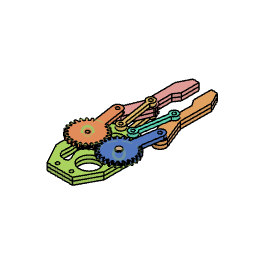
stage 3 v3 (Autodesk Fusion 360 design; units mm, degrees)
description: Spur Gear; Module: 1.125; Num Teeth: 24; Pressure Angle: 20.0; Backlash: 0.00 mm
Autodesk Fusion 360 part; units mm, degrees
note: some values were not read from the file. Chosen so that the rebuilt part matches the saved one: a direction. Set by a fixed rule: which sketch regions a step uses.
(part 1 of 6)
sketch "Sketch1" plane through (0, 0, 0) normal (0, 0, 1) x (1, 0, 0)
  line L0 (0, -5) -> (22, -5)
  arc A0 (22, -5) -> (22, 5) centre (22, 0) ccw
  line L1 (22, 5) -> (0, 5)
  arc A1 (0, 5) -> (0, -5) centre (0, 0) ccw
  line L2 (0, 0) -> (22, 0) construction
  circle A2 centre (0, 0) radius 1.5
  line L3 (20.05, 5) -> (54.05, 18.9791)
  line L4 (54.05, 18.9791) -> (57.9654, 9.456)
  line L5 (57.9654, 9.456) -> (23.1073, -4.8758)
  line L6 (44.6879, 15.1299) -> (56.0077, 14.2176)
  line L7 (43.85, 3.6525) -> (38, 5)
  line L8 (38, 5) -> (26.978, 0.4683)
  circle A3 centre (22, 0) radius 1.5
  dimension "d1" = 22
  dimension "d2" = 10
  dimension "d3" = 3
  dimension "d4" = 157.65
  dimension "d5" = 34
  dimension "d6" = 1.95
  dimension "d7" = 3
  constraint tangent L0 A0
  constraint tangent A0 L1
  constraint parallel L0 L1
  constraint tangent L1 A1
  constraint tangent L0 A1
  constraint horizontal L2
  constraint coincident A1.centre L2.start
  constraint coincident L1 L3.start
  constraint perpendicular L3 L4
  constraint coincident A0 L5.end
  constraint perpendicular L4 L5
  constraint coincident L3 L6.start
  constraint midpoint L4 L6.end
  constraint coincident L5 L7.start
  constraint coincident A0 L8.end
  constraint parallel L5 L8
  constraint concentric A0 A3
  measures "d1" distance of A1.centre A0.centre
  measures "d2" diameter of A1
  measures "d3" diameter of A2
  measures "d4" angle of L1 L3
  measures "d5" horizontal distance of L3.start L3.end
  measures "d6" horizontal distance of A0.centre L3.start
  measures "d7" diameter of A3
extrude "Extrude1" add sketch "Sketch1" along normal blind 3 contours L0 A0 L1 A1 L5 | A0 L1 L3 L4 L5 L6 L7 L8 makes body 1 in component "Component"
sketch "Sketch2" plane through (0, 0, 0) normal (0, 0, 1) x (1, 0, 0)
  circle A0 centre (75, 75) radius 1.5
  circle A1 centre (75, 75) radius 3.5
  circle A2 centre (106, 75) radius 3.5
  circle A3 centre (106, 75) radius 1.5
  line L0 (75, 75) -> (106, 75)
  line L1 (78.1623, 76.5) -> (102.8377, 76.5)
  line L2 (78.1623, 73.5) -> (102.8377, 73.5)
  dimension "d12" = 3
  dimension "d13" = 7
  dimension "d15" = 3
  dimension "d16" = 7
  dimension "d17" = 31
  dimension "d18" = 1.5
  constraint concentric A0 A1
  constraint concentric A2 A3
  constraint coincident A0.centre A1.centre
  constraint coincident A2.centre A3.centre
  constraint horizontal L0
  constraint coincident A1 L1.start
  constraint coincident A2 L1.end
  constraint parallel L0 L1
  constraint symmetric L0 L1.start L2.start
  constraint symmetric L0 L1.end L2.end
  measures "d12" diameter of A0
  measures "d13" diameter of A1
  measures "d15" diameter of A3
  measures "d16" diameter of A2
  measures "d17" distance of A0.centre A2.centre
  measures "d18" distance of L0 L1
extrude "Extrude1'" add sketch "Sketch2" along normal blind 3 separate body makes body 2 in component "Component'"
sketch "Sketch3" plane through (0, 0, 0) normal (0, 0, 1) x (1, 0, 0)
  line L0 (0, 0) -> (0, 62)
  line L1 (0, 62) -> (-7.9898, 62)
  line L2 (-7.9898, 62) -> (-20.5, 47.8997)
  line L3 (-20.5, 47.8997) -> (-20.5, 17.5997)
  line L4 (-20.5, 17.5997) -> (-11, 0)
  line L5 (-11, 0) -> (0, 0)
  circle A0 centre (-6, 4) radius 1.5
  circle A1 centre (-13.5, 37.5997) radius 1.5
  circle A2 centre (-5.2398, 58) radius 1.5
  line L6 (20.5, 17.5997) -> (11, 0)
  circle A3 centre (6, 4) radius 1.5
  circle A4 centre (13.5, 37.5997) radius 1.5
  line L7 (20.5, 47.8997) -> (20.5, 17.5997)
  circle A5 centre (5.2398, 58) radius 1.5
  line L8 (7.9898, 62) -> (20.5, 47.8997)
  line L9 (0, 62) -> (7.9898, 62)
  line L10 (11, 0) -> (0, 0)
  circle A6 centre (7.5, 17.691) radius 8.5
  line L11 (20.5, 17.5997) -> (0, 17.5997) construction
  dimension "d21" = 62
  dimension "d22" = 11
  dimension "d23" = 20
  dimension "d24" = 20.5
  dimension "d25" = 30.3
  dimension "d26" = 18.85
  dimension "d27" = 3
  dimension "d28" = 3
  dimension "d29" = 3
  dimension "d30" = 4
  dimension "d31" = 2.75
  dimension "d32" = 10.3
  dimension "d33" = 7
  dimension "d34" = 6
  dimension "d35" = 4
  dimension "d36" = 17
  dimension "d37" = 13
  constraint coincident L0.start L5.end
  constraint vertical L0
  constraint perpendicular L0 L1
  constraint perpendicular L1 L3
  constraint perpendicular L0 L5
  constraint symmetric L1.start L0 L9.start
  constraint symmetric L0 L1.end L8.start
  constraint symmetric L0 L2.end L7.start
  constraint symmetric L0 L3.end L6.start
  constraint symmetric L0 L4.end L6.end
  constraint symmetric L0 L5.end L10.end
  constraint symmetric L0 A0 A3
  constraint symmetric L0 A1 A4
  constraint symmetric L0 A2 A5
  constraint coincident L0 L11.end
  constraint perpendicular L0 L11
  measures "d21" distance of L0.start L0.end
  measures "d22" distance of L0.start L4.end
  measures "d23" distance of L3.end L4.end
  measures "d24" distance of L0 L3
  measures "d25" distance of L2.end L3.end
  measures "d26" distance of L1.end L2.end
  measures "d27" diameter of A0
  measures "d28" diameter of A1
  measures "d29" diameter of A2
  measures "d30" distance of L1 A2.centre
  measures "d31" horizontal distance of L1.end A2.centre
  measures "d32" vertical distance of L2.end A1.centre
  measures "d33" distance of L3 A1.centre
  measures "d34" distance of L0 A0.centre
  measures "d35" distance of L5 A0.centre
  measures "d36" diameter of A6
  measures "d37" distance of L7 A6.centre
extrude "Extrude1''" add sketch "Sketch3" along normal blind 3 separate body contours L0 L1 L2 L3 L4 L5 A6 | L0 L6 L7 L8 L9 L10 A6 makes body 3 in component "Component''"
sketch "Sketch4" plane through (0, 0, 3) normal (0, 0, 1) x (-1, 0, 0)
  circle A0 centre (-6, -4) radius 1.5
  circle A1 centre (5.2398, -58) radius 1.5
  circle A2 centre (-13.5, -37.5997) radius 1.5
  circle A3 centre (13.5, -37.5997) radius 1.5
  circle A4 centre (-5.2398, -58) radius 1.5
  circle A5 centre (-7.5, -17.691) radius 8.5
  circle A6 centre (6, -4) radius 1.5
  line L0 (-7.9898, -62) -> (7.9898, -62)
  line L1 (7.9898, -62) -> (20.5, -47.8997)
  line L2 (20.5, -47.8997) -> (20.5, -17.5997)
  line L3 (20.5, -17.5997) -> (11, 0)
  line L4 (11, 0) -> (-11, 0)
  line L5 (-11, 0) -> (-20.5, -17.5997)
  line L6 (-20.5, -17.5997) -> (-20.5, -47.8997)
  line L7 (-20.5, -47.8997) -> (-7.9898, -62)
  spline S0 degree 5 poles (12.8917, -32.7497) (13.0627, -32.4632) (13.3546, -31.885) (13.6389, -31.0021) (13.7288, -29.7898) (13.5064, -28.2005) (13.1435, -26.5229) (12.8276, -24.7511) (12.6826, -22.8957) (12.7202, -20.9894) (12.8744, -19.0806) (13.0281, -17.2268) (13.0445, -15.4879) (12.7941, -13.9207) (12.1875, -12.5709) (11.1918, -11.4723) (9.8351, -10.6528) (8.2144, -10.1372) (6.5032, -9.9521) (4.9542, -10.1289) (3.8249, -10.6926) (3.313, -11.651) (3.481, -12.9843) (4.2035, -14.636) (5.237, -16.5257) (6.2749, -18.5586) (7.0095, -20.6357) (7.187, -22.6645) (6.6764, -24.5697) (5.4931, -26.2997) (3.7541, -27.8255) (1.6495, -29.1413) (-0.5914, -30.2642) (-2.7325, -31.2346) (-4.564, -32.1163) (-5.9344, -32.9966) (-6.7579, -33.9688) (-7.023, -35.1132) (-6.7972, -36.4818) (-6.2425, -38.0755) (-5.5816, -39.8499) (-5.0441, -41.7334) (-4.8154, -43.6417) (-4.9903, -45.4931) (-5.5124, -47.2252) (-6.1547, -48.8042) (-6.6179, -50.2096) (-6.6131, -51.422) (-5.9409, -52.4113) (-4.5943, -53.121) (-2.7389, -53.4778) (-0.6363, -53.4144) (1.4172, -52.8895) (3.1524, -51.9058) (4.4015, -50.5363) (5.1121, -48.9126) (5.3227, -47.1881) (5.1507, -45.5081) (4.7735, -43.9799) (4.4175, -42.6349) (4.3186, -41.4371) (4.6666, -40.3184) (5.5597, -39.2036) (6.9404, -38.0442) (8.6243, -36.8193) (10.364, -35.5256) (11.5934, -34.4412) (12.3286, -33.6043) (12.7207, -33.0363) (12.8917, -32.7497) knots 0 0 0 0 0 0 0.01538462 0.03076923 0.04615385 0.06153846 0.07692308 0.09230769 0.10769231 0.12307692 0.13846154 0.15384615 0.16923077 0.18461538 0.2 0.21538462 0.23076923 0.24615385 0.26153846 0.27692308 0.29230769 0.30769231 0.32307692 0.33846154 0.35384615 0.36923077 0.38461538 0.4 0.41538462 0.43076923 0.44615385 0.46153846 0.47692308 0.49230769 0.50769231 0.52307692 0.53846154 0.55384615 0.56923077 0.58461538 0.6 0.61538462 0.63076923 0.64615385 0.66153846 0.67692308 0.69230769 0.70769231 0.72307692 0.73846154 0.75384615 0.76923077 0.78461538 0.8 0.81538462 0.83076923 0.84615385 0.86153846 0.87692308 0.89230769 0.90769231 0.92307692 0.93846154 0.95384615 0.96923077 0.98461538 1 1 1 1 1 1
  point P0 (12.8917, -24.9044)
  point P1 (12.8917, -14.7962)
  point P2 (8.3503, -10.2548)
  point P3 (3.5159, -11.5732)
  point P4 (7.0318, -21.828)
  point P5 (-2.6369, -31.2038)
  point P6 (-6.8853, -35.5987)
  point P7 (-5, -45)
  point P8 (-6.2994, -51.7133)
  point P9 (2.051, -52.4458)
  point P10 (5, -45)
  point P11 (5, -40)
extrude "Extrude2" cut sketch "Sketch4" against normal blind 3 contours S0 bodies 3 in component "Component''"
sketch "Sketch1 (2)" plane through (0, 0, 0) normal (0, 0, 1) x (1, 0, 0) in component "Spur Gear (24 teeth)"
  circle A0 centre (0, 0) radius 12.0992
  circle A1 centre (0, 0) radius 1.5
extrude "Extrude1'''" add sketch "Sketch1 (2)" along normal blind 3 separate body makes body 4 in component "Spur Gear (24 teeth)"
sketch "Sketch2 (2)" plane through (0, 0, 0) normal (0, 0, 1) x (1, 0, 0) in component "Spur Gear (24 teeth)"
  spline S0 degree 5 poles (12.6449, -1.0183) (12.6506, -1.0187) (12.6618, -1.0195) (12.6788, -1.0202) (12.7014, -1.0203) (12.7297, -1.0195) (12.758, -1.0178) (12.7864, -1.0156) (12.8147, -1.0131) (12.8431, -1.0105) (12.8715, -1.0076) (12.8999, -1.0045) (12.9284, -1.0011) (12.9568, -0.9973) (12.9852, -0.9932) (13.0137, -0.9886) (13.0421, -0.9838) (13.0705, -0.9787) (13.099, -0.9733) (13.1274, -0.9678) (13.1559, -0.962) (13.1843, -0.956) (13.2127, -0.9498) (13.2412, -0.9433) (13.2696, -0.9366) (13.298, -0.9297) (13.3264, -0.9226) (13.3549, -0.9152) (13.3833, -0.9076) (13.4117, -0.8999) (13.4401, -0.8919) (13.4684, -0.8838) (13.4968, -0.8754) (13.5252, -0.8669) (13.5535, -0.8581) (13.5819, -0.8492) (13.6102, -0.8401) (13.6385, -0.8308) (13.6669, -0.8214) (13.6952, -0.8117) (13.7234, -0.8019) (13.7517, -0.7919) (13.78, -0.7817) (13.8082, -0.7714) (13.8365, -0.7609) (13.8647, -0.7502) (13.8929, -0.7393) (13.9211, -0.7283) (13.9492, -0.7171) (13.9774, -0.7058) (14.0055, -0.6943) (14.0337, -0.6826) (14.0618, -0.6708) (14.0898, -0.6588) (14.1179, -0.6467) (14.146, -0.6344) (14.174, -0.6219) (14.202, -0.6093) (14.23, -0.5966) (14.2579, -0.5837) (14.2859, -0.5706) (14.3138, -0.5574) (14.3417, -0.544) (14.3696, -0.5305) (14.3975, -0.5169) (14.4253, -0.5031) (14.4531, -0.4891) (14.4809, -0.4751) (14.5087, -0.4608) (14.5364, -0.4465) (14.5641, -0.4319) (14.5863, -0.4202) (14.6029, -0.4114) (14.6139, -0.4054) (14.6195, -0.4024) knots 0 0 0 0 0 0 0.01428571 0.02857143 0.04285714 0.05714286 0.07142857 0.08571429 0.1 0.11428571 0.12857143 0.14285714 0.15714286 0.17142857 0.18571429 0.2 0.21428571 0.22857143 0.24285714 0.25714286 0.27142857 0.28571429 0.3 0.31428571 0.32857143 0.34285714 0.35714286 0.37142857 0.38571429 0.4 0.41428571 0.42857143 0.44285714 0.45714286 0.47142857 0.48571429 0.5 0.51428571 0.52857143 0.54285714 0.55714286 0.57142857 0.58571429 0.6 0.61428571 0.62857143 0.64285714 0.65714286 0.67142857 0.68571429 0.7 0.71428571 0.72857143 0.74285714 0.75714286 0.77142857 0.78571429 0.8 0.81428571 0.82857143 0.84285714 0.85714286 0.87142857 0.88571429 0.9 0.91428571 0.92857143 0.94285714 0.95714286 0.97142857 0.98571429 1 1 1 1 1 1
  spline S1 degree 5 poles (12.6449, 1.0183) (12.6506, 1.0187) (12.6618, 1.0195) (12.6788, 1.0202) (12.7014, 1.0203) (12.7297, 1.0195) (12.758, 1.0178) (12.7864, 1.0156) (12.8147, 1.0131) (12.8431, 1.0105) (12.8715, 1.0076) (12.8999, 1.0045) (12.9284, 1.0011) (12.9568, 0.9973) (12.9852, 0.9932) (13.0137, 0.9886) (13.0421, 0.9838) (13.0705, 0.9787) (13.099, 0.9733) (13.1274, 0.9678) (13.1559, 0.962) (13.1843, 0.956) (13.2127, 0.9498) (13.2412, 0.9433) (13.2696, 0.9366) (13.298, 0.9297) (13.3264, 0.9226) (13.3549, 0.9152) (13.3833, 0.9076) (13.4117, 0.8999) (13.4401, 0.8919) (13.4684, 0.8838) (13.4968, 0.8754) (13.5252, 0.8669) (13.5535, 0.8581) (13.5819, 0.8492) (13.6102, 0.8401) (13.6385, 0.8308) (13.6669, 0.8214) (13.6952, 0.8117) (13.7234, 0.8019) (13.7517, 0.7919) (13.78, 0.7817) (13.8082, 0.7714) (13.8365, 0.7609) (13.8647, 0.7502) (13.8929, 0.7393) (13.9211, 0.7283) (13.9492, 0.7171) (13.9774, 0.7058) (14.0055, 0.6943) (14.0337, 0.6826) (14.0618, 0.6708) (14.0898, 0.6588) (14.1179, 0.6467) (14.146, 0.6344) (14.174, 0.6219) (14.202, 0.6093) (14.23, 0.5966) (14.2579, 0.5837) (14.2859, 0.5706) (14.3138, 0.5574) (14.3417, 0.544) (14.3696, 0.5305) (14.3975, 0.5169) (14.4253, 0.5031) (14.4531, 0.4891) (14.4809, 0.4751) (14.5087, 0.4608) (14.5364, 0.4465) (14.5641, 0.4319) (14.5863, 0.4202) (14.6029, 0.4114) (14.6139, 0.4054) (14.6195, 0.4024) knots 0 0 0 0 0 0 0.01428571 0.02857143 0.04285714 0.05714286 0.07142857 0.08571429 0.1 0.11428571 0.12857143 0.14285714 0.15714286 0.17142857 0.18571429 0.2 0.21428571 0.22857143 0.24285714 0.25714286 0.27142857 0.28571429 0.3 0.31428571 0.32857143 0.34285714 0.35714286 0.37142857 0.38571429 0.4 0.41428571 0.42857143 0.44285714 0.45714286 0.47142857 0.48571429 0.5 0.51428571 0.52857143 0.54285714 0.55714286 0.57142857 0.58571429 0.6 0.61428571 0.62857143 0.64285714 0.65714286 0.67142857 0.68571429 0.7 0.71428571 0.72857143 0.74285714 0.75714286 0.77142857 0.78571429 0.8 0.81428571 0.82857143 0.84285714 0.85714286 0.87142857 0.88571429 0.9 0.91428571 0.92857143 0.94285714 0.95714286 0.97142857 0.98571429 1 1 1 1 1 1
  arc A0 (14.6195, -0.4024) -> (14.6195, 0.4024) centre (0, 0) ccw
  line L0 (12.0502, -0.9712) -> (12.6449, -1.0183)
  line L1 (12.0502, 0.9712) -> (12.6449, 1.0183)
  line L2 (12.0502, -0.9712) -> (12.0502, 0.9712)
  point P0 (12.7841, -1.0157)
  point P1 (12.9241, -1.0016)
  point P2 (13.0647, -0.9797)
  point P3 (13.2057, -0.9513)
  point P4 (13.3469, -0.9172)
  point P5 (13.4884, -0.8779)
  point P6 (13.63, -0.8336)
  point P7 (13.7716, -0.7847)
  point P8 (13.9132, -0.7313)
  point P9 (14.0548, -0.6737)
  point P10 (14.1963, -0.6119)
  point P11 (14.3376, -0.546)
  point P12 (14.4787, -0.4761)
  point P13 (12.7841, 1.0157)
  point P14 (12.9241, 1.0016)
  point P15 (13.0647, 0.9797)
  point P16 (13.2057, 0.9513)
  point P17 (13.3469, 0.9172)
  point P18 (13.4884, 0.8779)
  point P19 (13.63, 0.8336)
  point P20 (13.7716, 0.7847)
  point P21 (13.9132, 0.7313)
  point P22 (14.0548, 0.6737)
  point P23 (14.1963, 0.6119)
  point P24 (14.3376, 0.546)
  point P25 (14.4787, 0.4761)
extrude "Extrude2'" add sketch "Sketch2 (2)" along normal blind 3 bodies 4 in component "Spur Gear (24 teeth)"
fillet "Fillet1" radius 0.1 2 edges at (12.0601, -0.972, 1.5) (12.0601, 0.972, 1.5) on bodies 4 in component "Spur Gear (24 teeth)"
pattern_circular "C-Pattern1" count 24 over 360 about axis through (0, 0, 0) along (0, 0, 1) of "Extrude2'", "Fillet1" in component "Spur Gear (24 teeth)"
sketch "Sketch3 (2)" plane through (0, 0, 0) normal (0, 0, 1) x (1, 0, 0) in component "Spur Gear (24 teeth)"
  circle A0 centre (0, 0) radius 13.5 construction
sketch "Sketch1 (3)" plane through (0, 0, 0) normal (0, 0, 1) x (1, 0, 0) in component "Spur Gear (24 teeth) (1)"
  circle A0 centre (0, 0) radius 12.0992
  circle A1 centre (0, 0) radius 1.5
extrude "Extrude1''''" add sketch "Sketch1 (3)" along normal blind 3 separate body makes body 5 in component "Spur Gear (24 teeth) (1)"
sketch "Sketch2 (3)" plane through (0, 0, 0) normal (0, 0, 1) x (1, 0, 0) in component "Spur Gear (24 teeth) (1)"
  spline S0 degree 5 poles (12.6449, -1.0183) (12.6506, -1.0187) (12.6618, -1.0195) (12.6788, -1.0202) (12.7014, -1.0203) (12.7297, -1.0195) (12.758, -1.0178) (12.7864, -1.0156) (12.8147, -1.0131) (12.8431, -1.0105) (12.8715, -1.0076) (12.8999, -1.0045) (12.9284, -1.0011) (12.9568, -0.9973) (12.9852, -0.9932) (13.0137, -0.9886) (13.0421, -0.9838) (13.0705, -0.9787) (13.099, -0.9733) (13.1274, -0.9678) (13.1559, -0.962) (13.1843, -0.956) (13.2127, -0.9498) (13.2412, -0.9433) (13.2696, -0.9366) (13.298, -0.9297) (13.3264, -0.9226) (13.3549, -0.9152) (13.3833, -0.9076) (13.4117, -0.8999) (13.4401, -0.8919) (13.4684, -0.8838) (13.4968, -0.8754) (13.5252, -0.8669) (13.5535, -0.8581) (13.5819, -0.8492) (13.6102, -0.8401) (13.6385, -0.8308) (13.6669, -0.8214) (13.6952, -0.8117) (13.7234, -0.8019) (13.7517, -0.7919) (13.78, -0.7817) (13.8082, -0.7714) (13.8365, -0.7609) (13.8647, -0.7502) (13.8929, -0.7393) (13.9211, -0.7283) (13.9492, -0.7171) (13.9774, -0.7058) (14.0055, -0.6943) (14.0337, -0.6826) (14.0618, -0.6708) (14.0898, -0.6588) (14.1179, -0.6467) (14.146, -0.6344) (14.174, -0.6219) (14.202, -0.6093) (14.23, -0.5966) (14.2579, -0.5837) (14.2859, -0.5706) (14.3138, -0.5574) (14.3417, -0.544) (14.3696, -0.5305) (14.3975, -0.5169) (14.4253, -0.5031) (14.4531, -0.4891) (14.4809, -0.4751) (14.5087, -0.4608) (14.5364, -0.4465) (14.5641, -0.4319) (14.5863, -0.4202) (14.6029, -0.4114) (14.6139, -0.4054) (14.6195, -0.4024) knots 0 0 0 0 0 0 0.01428571 0.02857143 0.04285714 0.05714286 0.07142857 0.08571429 0.1 0.11428571 0.12857143 0.14285714 0.15714286 0.17142857 0.18571429 0.2 0.21428571 0.22857143 0.24285714 0.25714286 0.27142857 0.28571429 0.3 0.31428571 0.32857143 0.34285714 0.35714286 0.37142857 0.38571429 0.4 0.41428571 0.42857143 0.44285714 0.45714286 0.47142857 0.48571429 0.5 0.51428571 0.52857143 0.54285714 0.55714286 0.57142857 0.58571429 0.6 0.61428571 0.62857143 0.64285714 0.65714286 0.67142857 0.68571429 0.7 0.71428571 0.72857143 0.74285714 0.75714286 0.77142857 0.78571429 0.8 0.81428571 0.82857143 0.84285714 0.85714286 0.87142857 0.88571429 0.9 0.91428571 0.92857143 0.94285714 0.95714286 0.97142857 0.98571429 1 1 1 1 1 1
  spline S1 degree 5 poles (12.6449, 1.0183) (12.6506, 1.0187) (12.6618, 1.0195) (12.6788, 1.0202) (12.7014, 1.0203) (12.7297, 1.0195) (12.758, 1.0178) (12.7864, 1.0156) (12.8147, 1.0131) (12.8431, 1.0105) (12.8715, 1.0076) (12.8999, 1.0045) (12.9284, 1.0011) (12.9568, 0.9973) (12.9852, 0.9932) (13.0137, 0.9886) (13.0421, 0.9838) (13.0705, 0.9787) (13.099, 0.9733) (13.1274, 0.9678) (13.1559, 0.962) (13.1843, 0.956) (13.2127, 0.9498) (13.2412, 0.9433) (13.2696, 0.9366) (13.298, 0.9297) (13.3264, 0.9226) (13.3549, 0.9152) (13.3833, 0.9076) (13.4117, 0.8999) (13.4401, 0.8919) (13.4684, 0.8838) (13.4968, 0.8754) (13.5252, 0.8669) (13.5535, 0.8581) (13.5819, 0.8492) (13.6102, 0.8401) (13.6385, 0.8308) (13.6669, 0.8214) (13.6952, 0.8117) (13.7234, 0.8019) (13.7517, 0.7919) (13.78, 0.7817) (13.8082, 0.7714) (13.8365, 0.7609) (13.8647, 0.7502) (13.8929, 0.7393) (13.9211, 0.7283) (13.9492, 0.7171) (13.9774, 0.7058) (14.0055, 0.6943) (14.0337, 0.6826) (14.0618, 0.6708) (14.0898, 0.6588) (14.1179, 0.6467) (14.146, 0.6344) (14.174, 0.6219) (14.202, 0.6093) (14.23, 0.5966) (14.2579, 0.5837) (14.2859, 0.5706) (14.3138, 0.5574) (14.3417, 0.544) (14.3696, 0.5305) (14.3975, 0.5169) (14.4253, 0.5031) (14.4531, 0.4891) (14.4809, 0.4751) (14.5087, 0.4608) (14.5364, 0.4465) (14.5641, 0.4319) (14.5863, 0.4202) (14.6029, 0.4114) (14.6139, 0.4054) (14.6195, 0.4024) knots 0 0 0 0 0 0 0.01428571 0.02857143 0.04285714 0.05714286 0.07142857 0.08571429 0.1 0.11428571 0.12857143 0.14285714 0.15714286 0.17142857 0.18571429 0.2 0.21428571 0.22857143 0.24285714 0.25714286 0.27142857 0.28571429 0.3 0.31428571 0.32857143 0.34285714 0.35714286 0.37142857 0.38571429 0.4 0.41428571 0.42857143 0.44285714 0.45714286 0.47142857 0.48571429 0.5 0.51428571 0.52857143 0.54285714 0.55714286 0.57142857 0.58571429 0.6 0.61428571 0.62857143 0.64285714 0.65714286 0.67142857 0.68571429 0.7 0.71428571 0.72857143 0.74285714 0.75714286 0.77142857 0.78571429 0.8 0.81428571 0.82857143 0.84285714 0.85714286 0.87142857 0.88571429 0.9 0.91428571 0.92857143 0.94285714 0.95714286 0.97142857 0.98571429 1 1 1 1 1 1
  arc A0 (14.6195, -0.4024) -> (14.6195, 0.4024) centre (0, 0) ccw
  line L0 (12.0502, -0.9712) -> (12.6449, -1.0183)
  line L1 (12.0502, 0.9712) -> (12.6449, 1.0183)
  line L2 (12.0502, -0.9712) -> (12.0502, 0.9712)
  point P0 (12.7841, -1.0157)
  point P1 (12.9241, -1.0016)
  point P2 (13.0647, -0.9797)
  point P3 (13.2057, -0.9513)
  point P4 (13.3469, -0.9172)
  point P5 (13.4884, -0.8779)
  point P6 (13.63, -0.8336)
  point P7 (13.7716, -0.7847)
  point P8 (13.9132, -0.7313)
  point P9 (14.0548, -0.6737)
  point P10 (14.1963, -0.6119)
  point P11 (14.3376, -0.546)
  point P12 (14.4787, -0.4761)
  point P13 (12.7841, 1.0157)
  point P14 (12.9241, 1.0016)
  point P15 (13.0647, 0.9797)
  point P16 (13.2057, 0.9513)
  point P17 (13.3469, 0.9172)
  point P18 (13.4884, 0.8779)
  point P19 (13.63, 0.8336)
  point P20 (13.7716, 0.7847)
  point P21 (13.9132, 0.7313)
  point P22 (14.0548, 0.6737)
  point P23 (14.1963, 0.6119)
  point P24 (14.3376, 0.546)
  point P25 (14.4787, 0.4761)
extrude "Extrude2''" add sketch "Sketch2 (3)" along normal blind 3 bodies 5 in component "Spur Gear (24 teeth) (1)"
fillet "Fillet1'" radius 0.1 2 edges at (12.0601, -0.972, 1.5) (12.0601, 0.972, 1.5) on bodies 5 in component "Spur Gear (24 teeth) (1)"
pattern_circular "C-Pattern1'" count 24 over 360 about axis through (0, 0, 0) along (0, 0, 1) of "Extrude2''", "Fillet1'" in component "Spur Gear (24 teeth) (1)"
sketch "Sketch3 (3)" plane through (0, 0, 0) normal (0, 0, 1) x (1, 0, 0) in component "Spur Gear (24 teeth) (1)"
  circle A0 centre (0, 0) radius 13.5 construction
sketch "Sketch5" plane through (0, 0, 6) normal (0, 0, 1) x (-1, 0, 0)
  circle A0 centre (13.5, -37.5997) radius 1.5
  arc A1 (8.1767, -48.5756) -> (8.1311, -48.4425) centre (8.0867, -48.5321) ccw
  line L0 (8.1767, -48.5756) -> (7.9648, -49.0143)
  spline S0 degree 5 poles (7.9648, -49.0143) (7.9623, -49.0194) (7.9575, -49.0296) (7.9507, -49.0451) (7.9423, -49.0661) (7.9329, -49.0928) (7.9242, -49.1198) (7.9159, -49.1471) (7.9079, -49.1744) (7.9001, -49.2018) (7.8925, -49.2293) (7.885, -49.2569) (7.8779, -49.2846) (7.8711, -49.3125) (7.8647, -49.3405) (7.8586, -49.3686) (7.8528, -49.3969) (7.8473, -49.4253) (7.842, -49.4537) (7.8368, -49.4822) (7.8319, -49.5108) (7.8271, -49.5395) (7.8226, -49.5682) (7.8183, -49.5971) (7.8143, -49.626) (7.8104, -49.655) (7.8068, -49.6841) (7.8033, -49.7132) (7.8001, -49.7425) (7.797, -49.7717) (7.7941, -49.8011) (7.7914, -49.8305) (7.7889, -49.86) (7.7866, -49.8895) (7.7844, -49.9191) (7.7824, -49.9487) (7.7807, -49.9784) (7.779, -50.0082) (7.7776, -50.038) (7.7763, -50.0679) (7.7752, -50.0978) (7.7743, -50.1278) (7.7735, -50.1578) (7.7729, -50.1879) (7.7725, -50.218) (7.7722, -50.2482) (7.7721, -50.2784) (7.7721, -50.3087) (7.7723, -50.339) (7.7727, -50.3693) (7.7732, -50.3997) (7.7739, -50.4302) (7.7747, -50.4607) (7.7757, -50.4912) (7.7768, -50.5217) (7.7781, -50.5523) (7.7795, -50.583) (7.7811, -50.6136) (7.7828, -50.6443) (7.7847, -50.6751) (7.7868, -50.7059) (7.7889, -50.7367) (7.7913, -50.7675) (7.7937, -50.7984) (7.7964, -50.8293) (7.7991, -50.8603) (7.802, -50.8912) (7.8051, -50.9222) (7.8083, -50.9533) (7.8116, -50.9843) (7.8151, -51.0154) (7.818, -51.0403) (7.8202, -51.059) (7.8217, -51.0715) (7.8225, -51.0777) knots 0 0 0 0 0 0 0.01428571 0.02857143 0.04285714 0.05714286 0.07142857 0.08571429 0.1 0.11428571 0.12857143 0.14285714 0.15714286 0.17142857 0.18571429 0.2 0.21428571 0.22857143 0.24285714 0.25714286 0.27142857 0.28571429 0.3 0.31428571 0.32857143 0.34285714 0.35714286 0.37142857 0.38571429 0.4 0.41428571 0.42857143 0.44285714 0.45714286 0.47142857 0.48571429 0.5 0.51428571 0.52857143 0.54285714 0.55714286 0.57142857 0.58571429 0.6 0.61428571 0.62857143 0.64285714 0.65714286 0.67142857 0.68571429 0.7 0.71428571 0.72857143 0.74285714 0.75714286 0.77142857 0.78571429 0.8 0.81428571 0.82857143 0.84285714 0.85714286 0.87142857 0.88571429 0.9 0.91428571 0.92857143 0.94285714 0.95714286 0.97142857 0.98571429 1 1 1 1 1 1
  arc A2 (7.8225, -51.0777) -> (8.5726, -51.3696) centre (13.5, -37.5997) ccw
  spline S1 degree 5 poles (9.8626, -49.7529) (9.861, -49.7583) (9.8576, -49.7691) (9.8521, -49.7852) (9.8441, -49.8063) (9.833, -49.8323) (9.8211, -49.8581) (9.8088, -49.8838) (9.7962, -49.9093) (9.7834, -49.9348) (9.7705, -49.9602) (9.7573, -49.9856) (9.7438, -50.0108) (9.73, -50.036) (9.7158, -50.0609) (9.7012, -50.0858) (9.6864, -50.1105) (9.6713, -50.1352) (9.656, -50.1597) (9.6405, -50.1842) (9.6249, -50.2087) (9.609, -50.233) (9.5929, -50.2572) (9.5765, -50.2814) (9.56, -50.3054) (9.5432, -50.3294) (9.5262, -50.3533) (9.5091, -50.3771) (9.4917, -50.4008) (9.4742, -50.4245) (9.4565, -50.4481) (9.4386, -50.4716) (9.4205, -50.495) (9.4023, -50.5183) (9.3838, -50.5416) (9.3652, -50.5648) (9.3465, -50.5879) (9.3275, -50.6109) (9.3084, -50.6338) (9.2892, -50.6567) (9.2698, -50.6795) (9.2502, -50.7022) (9.2305, -50.7249) (9.2106, -50.7475) (9.1905, -50.77) (9.1704, -50.7924) (9.15, -50.8147) (9.1295, -50.837) (9.1089, -50.8592) (9.0881, -50.8813) (9.0672, -50.9034) (9.0461, -50.9253) (9.0249, -50.9472) (9.0035, -50.9691) (8.9821, -50.9908) (8.9604, -51.0125) (8.9387, -51.0341) (8.9168, -51.0556) (8.8947, -51.0771) (8.8725, -51.0985) (8.8502, -51.1198) (8.8278, -51.141) (8.8052, -51.1622) (8.7825, -51.1832) (8.7597, -51.2043) (8.7368, -51.2252) (8.7137, -51.2461) (8.6905, -51.2668) (8.6671, -51.2876) (8.6437, -51.3082) (8.6201, -51.3288) (8.6011, -51.3451) (8.5869, -51.3574) (8.5773, -51.3656) (8.5726, -51.3696) knots 0 0 0 0 0 0 0.01428571 0.02857143 0.04285714 0.05714286 0.07142857 0.08571429 0.1 0.11428571 0.12857143 0.14285714 0.15714286 0.17142857 0.18571429 0.2 0.21428571 0.22857143 0.24285714 0.25714286 0.27142857 0.28571429 0.3 0.31428571 0.32857143 0.34285714 0.35714286 0.37142857 0.38571429 0.4 0.41428571 0.42857143 0.44285714 0.45714286 0.47142857 0.48571429 0.5 0.51428571 0.52857143 0.54285714 0.55714286 0.57142857 0.58571429 0.6 0.61428571 0.62857143 0.64285714 0.65714286 0.67142857 0.68571429 0.7 0.71428571 0.72857143 0.74285714 0.75714286 0.77142857 0.78571429 0.8 0.81428571 0.82857143 0.84285714 0.85714286 0.87142857 0.88571429 0.9 0.91428571 0.92857143 0.94285714 0.95714286 0.97142857 0.98571429 1 1 1 1 1 1
  line L1 (9.8626, -49.7529) -> (10.0029, -49.2864)
  arc A3 (10.1266, -49.2191) -> (10.0029, -49.2864) centre (10.0987, -49.3152) ccw
  arc A4 (10.1266, -49.2191) -> (11.1203, -49.4626) centre (13.5, -37.5997) ccw
  arc A5 (11.1989, -49.5794) -> (11.1203, -49.4626) centre (11.1007, -49.5606) ccw
  line L2 (11.1989, -49.5794) -> (11.1077, -50.0579)
  spline S2 degree 5 poles (11.1077, -50.0579) (11.1066, -50.0635) (11.1046, -50.0746) (11.1021, -50.0914) (11.0994, -50.1139) (11.0972, -50.1421) (11.0958, -50.1704) (11.0949, -50.1989) (11.0942, -50.2273) (11.0938, -50.2558) (11.0935, -50.2844) (11.0935, -50.313) (11.0938, -50.3416) (11.0944, -50.3702) (11.0955, -50.399) (11.0969, -50.4277) (11.0986, -50.4565) (11.1006, -50.4853) (11.1028, -50.5142) (11.1052, -50.5431) (11.1078, -50.572) (11.1107, -50.6009) (11.1137, -50.6298) (11.1171, -50.6588) (11.1206, -50.6878) (11.1244, -50.7168) (11.1284, -50.7458) (11.1326, -50.7749) (11.1371, -50.804) (11.1417, -50.833) (11.1465, -50.8621) (11.1515, -50.8912) (11.1567, -50.9203) (11.1621, -50.9495) (11.1677, -50.9786) (11.1734, -51.0078) (11.1794, -51.0369) (11.1855, -51.0661) (11.1919, -51.0953) (11.1984, -51.1245) (11.205, -51.1536) (11.2119, -51.1828) (11.2189, -51.212) (11.2261, -51.2413) (11.2335, -51.2705) (11.241, -51.2997) (11.2487, -51.3289) (11.2566, -51.3581) (11.2646, -51.3873) (11.2728, -51.4166) (11.2812, -51.4458) (11.2897, -51.475) (11.2984, -51.5042) (11.3073, -51.5335) (11.3163, -51.5627) (11.3254, -51.5919) (11.3347, -51.6211) (11.3442, -51.6503) (11.3538, -51.6796) (11.3636, -51.7088) (11.3735, -51.738) (11.3836, -51.7672) (11.3939, -51.7964) (11.4042, -51.8256) (11.4148, -51.8547) (11.4254, -51.8839) (11.4363, -51.9131) (11.4472, -51.9422) (11.4584, -51.9714) (11.4696, -52.0005) (11.481, -52.0297) (11.4903, -52.053) (11.4972, -52.0704) (11.5019, -52.0821) (11.5043, -52.0879) knots 0 0 0 0 0 0 0.01428571 0.02857143 0.04285714 0.05714286 0.07142857 0.08571429 0.1 0.11428571 0.12857143 0.14285714 0.15714286 0.17142857 0.18571429 0.2 0.21428571 0.22857143 0.24285714 0.25714286 0.27142857 0.28571429 0.3 0.31428571 0.32857143 0.34285714 0.35714286 0.37142857 0.38571429 0.4 0.41428571 0.42857143 0.44285714 0.45714286 0.47142857 0.48571429 0.5 0.51428571 0.52857143 0.54285714 0.55714286 0.57142857 0.58571429 0.6 0.61428571 0.62857143 0.64285714 0.65714286 0.67142857 0.68571429 0.7 0.71428571 0.72857143 0.74285714 0.75714286 0.77142857 0.78571429 0.8 0.81428571 0.82857143 0.84285714 0.85714286 0.87142857 0.88571429 0.9 0.91428571 0.92857143 0.94285714 0.95714286 0.97142857 0.98571429 1 1 1 1 1 1
  arc A6 (11.5043, -52.0879) -> (12.3044, -52.1758) centre (13.5, -37.5997) ccw
  spline S3 degree 5 poles (13.132, -50.2802) (13.1319, -50.2859) (13.1314, -50.2972) (13.1302, -50.3141) (13.1279, -50.3366) (13.124, -50.3646) (13.1192, -50.3926) (13.1139, -50.4205) (13.1084, -50.4485) (13.1026, -50.4764) (13.0967, -50.5043) (13.0905, -50.5322) (13.0841, -50.5601) (13.0772, -50.588) (13.0699, -50.6158) (13.0623, -50.6435) (13.0544, -50.6713) (13.0462, -50.699) (13.0378, -50.7267) (13.0292, -50.7543) (13.0203, -50.782) (13.0113, -50.8096) (13.002, -50.8372) (12.9925, -50.8647) (12.9827, -50.8923) (12.9727, -50.9198) (12.9625, -50.9472) (12.9521, -50.9747) (12.9415, -51.0021) (12.9306, -51.0295) (12.9196, -51.0568) (12.9084, -51.0841) (12.897, -51.1114) (12.8855, -51.1387) (12.8737, -51.1659) (12.8617, -51.1931) (12.8496, -51.2203) (12.8373, -51.2475) (12.8247, -51.2746) (12.8121, -51.3016) (12.7992, -51.3287) (12.7862, -51.3557) (12.773, -51.3827) (12.7596, -51.4096) (12.7461, -51.4366) (12.7324, -51.4634) (12.7185, -51.4903) (12.7045, -51.5171) (12.6903, -51.5439) (12.676, -51.5706) (12.6615, -51.5974) (12.6468, -51.624) (12.632, -51.6507) (12.617, -51.6773) (12.6019, -51.7039) (12.5866, -51.7304) (12.5712, -51.7569) (12.5556, -51.7834) (12.5398, -51.8098) (12.524, -51.8362) (12.5079, -51.8625) (12.4917, -51.8888) (12.4754, -51.9151) (12.459, -51.9414) (12.4424, -51.9676) (12.4256, -51.9937) (12.4087, -52.0199) (12.3917, -52.0459) (12.3745, -52.072) (12.3572, -52.098) (12.3397, -52.124) (12.3257, -52.1447) (12.315, -52.1602) (12.3079, -52.1706) (12.3044, -52.1758) knots 0 0 0 0 0 0 0.01428571 0.02857143 0.04285714 0.05714286 0.07142857 0.08571429 0.1 0.11428571 0.12857143 0.14285714 0.15714286 0.17142857 0.18571429 0.2 0.21428571 0.22857143 0.24285714 0.25714286 0.27142857 0.28571429 0.3 0.31428571 0.32857143 0.34285714 0.35714286 0.37142857 0.38571429 0.4 0.41428571 0.42857143 0.44285714 0.45714286 0.47142857 0.48571429 0.5 0.51428571 0.52857143 0.54285714 0.55714286 0.57142857 0.58571429 0.6 0.61428571 0.62857143 0.64285714 0.65714286 0.67142857 0.68571429 0.7 0.71428571 0.72857143 0.74285714 0.75714286 0.77142857 0.78571429 0.8 0.81428571 0.82857143 0.84285714 0.85714286 0.87142857 0.88571429 0.9 0.91428571 0.92857143 0.94285714 0.95714286 0.97142857 0.98571429 1 1 1 1 1 1
  line L3 (13.132, -50.2802) -> (13.1468, -49.7933)
  arc A7 (13.2488, -49.6963) -> (13.1468, -49.7933) centre (13.2468, -49.7963) ccw
  arc A8 (13.2488, -49.6963) -> (14.2718, -49.6743) centre (13.5, -37.5997) ccw
  arc A9 (14.3779, -49.7667) -> (14.2718, -49.6743) centre (14.2781, -49.7741) ccw
  line L4 (14.3779, -49.7667) -> (14.4136, -50.2526)
  spline S4 degree 5 poles (14.4136, -50.2526) (14.414, -50.2583) (14.415, -50.2695) (14.4169, -50.2864) (14.4201, -50.3088) (14.4253, -50.3366) (14.4313, -50.3643) (14.4377, -50.392) (14.4445, -50.4197) (14.4514, -50.4474) (14.4585, -50.475) (14.4659, -50.5026) (14.4736, -50.5302) (14.4817, -50.5577) (14.4901, -50.5852) (14.4989, -50.6126) (14.508, -50.64) (14.5174, -50.6673) (14.527, -50.6946) (14.5368, -50.7219) (14.5468, -50.7491) (14.557, -50.7763) (14.5675, -50.8035) (14.5782, -50.8306) (14.5891, -50.8577) (14.6003, -50.8847) (14.6117, -50.9117) (14.6233, -50.9387) (14.6351, -50.9656) (14.6471, -50.9925) (14.6592, -51.0194) (14.6716, -51.0462) (14.6842, -51.073) (14.6969, -51.0997) (14.7098, -51.1264) (14.723, -51.1531) (14.7363, -51.1797) (14.7498, -51.2063) (14.7634, -51.2328) (14.7772, -51.2593) (14.7912, -51.2858) (14.8054, -51.3122) (14.8198, -51.3386) (14.8343, -51.365) (14.849, -51.3913) (14.8638, -51.4175) (14.8788, -51.4438) (14.894, -51.47) (14.9093, -51.4961) (14.9248, -51.5222) (14.9404, -51.5483) (14.9562, -51.5743) (14.9722, -51.6003) (14.9883, -51.6262) (15.0046, -51.6521) (15.021, -51.678) (15.0375, -51.7038) (15.0542, -51.7295) (15.0711, -51.7553) (15.0881, -51.781) (15.1053, -51.8066) (15.1226, -51.8322) (15.14, -51.8577) (15.1576, -51.8832) (15.1753, -51.9087) (15.1932, -51.9341) (15.2112, -51.9595) (15.2293, -51.9848) (15.2476, -52.0101) (15.266, -52.0353) (15.2846, -52.0605) (15.2995, -52.0806) (15.3108, -52.0957) (15.3183, -52.1057) (15.3221, -52.1108) knots 0 0 0 0 0 0 0.01428571 0.02857143 0.04285714 0.05714286 0.07142857 0.08571429 0.1 0.11428571 0.12857143 0.14285714 0.15714286 0.17142857 0.18571429 0.2 0.21428571 0.22857143 0.24285714 0.25714286 0.27142857 0.28571429 0.3 0.31428571 0.32857143 0.34285714 0.35714286 0.37142857 0.38571429 0.4 0.41428571 0.42857143 0.44285714 0.45714286 0.47142857 0.48571429 0.5 0.51428571 0.52857143 0.54285714 0.55714286 0.57142857 0.58571429 0.6 0.61428571 0.62857143 0.64285714 0.65714286 0.67142857 0.68571429 0.7 0.71428571 0.72857143 0.74285714 0.75714286 0.77142857 0.78571429 0.8 0.81428571 0.82857143 0.84285714 0.85714286 0.87142857 0.88571429 0.9 0.91428571 0.92857143 0.94285714 0.95714286 0.97142857 0.98571429 1 1 1 1 1 1
  arc A10 (15.3221, -52.1108) -> (16.1177, -51.9885) centre (13.5, -37.5997) ccw
  spline S5 degree 5 poles (16.4265, -49.9434) (16.4278, -49.9489) (16.4303, -49.9599) (16.4336, -49.9766) (16.4371, -49.9989) (16.4406, -50.027) (16.4432, -50.0553) (16.4454, -50.0836) (16.4472, -50.112) (16.4489, -50.1405) (16.4504, -50.169) (16.4517, -50.1975) (16.4526, -50.2262) (16.4532, -50.2548) (16.4534, -50.2836) (16.4532, -50.3124) (16.4527, -50.3412) (16.452, -50.3701) (16.451, -50.399) (16.4499, -50.428) (16.4485, -50.4569) (16.4469, -50.486) (16.4451, -50.515) (16.443, -50.5441) (16.4407, -50.5732) (16.4382, -50.6024) (16.4354, -50.6315) (16.4324, -50.6607) (16.4293, -50.69) (16.4259, -50.7192) (16.4224, -50.7485) (16.4186, -50.7778) (16.4147, -50.8071) (16.4106, -50.8364) (16.4062, -50.8658) (16.4017, -50.8952) (16.397, -50.9245) (16.3921, -50.954) (16.3871, -50.9834) (16.3818, -51.0128) (16.3764, -51.0423) (16.3708, -51.0717) (16.3651, -51.1012) (16.3591, -51.1307) (16.353, -51.1602) (16.3467, -51.1897) (16.3403, -51.2192) (16.3337, -51.2488) (16.3269, -51.2783) (16.32, -51.3079) (16.3129, -51.3374) (16.3056, -51.367) (16.2982, -51.3966) (16.2906, -51.4261) (16.2829, -51.4557) (16.275, -51.4853) (16.267, -51.5149) (16.2587, -51.5445) (16.2504, -51.5741) (16.2419, -51.6037) (16.2332, -51.6333) (16.2244, -51.6629) (16.2154, -51.6925) (16.2063, -51.7221) (16.1971, -51.7517) (16.1877, -51.7813) (16.1781, -51.8109) (16.1684, -51.8406) (16.1585, -51.8702) (16.1486, -51.8998) (16.1384, -51.9294) (16.1302, -51.953) (16.124, -51.9708) (16.1198, -51.9826) (16.1177, -51.9885) knots 0 0 0 0 0 0 0.01428571 0.02857143 0.04285714 0.05714286 0.07142857 0.08571429 0.1 0.11428571 0.12857143 0.14285714 0.15714286 0.17142857 0.18571429 0.2 0.21428571 0.22857143 0.24285714 0.25714286 0.27142857 0.28571429 0.3 0.31428571 0.32857143 0.34285714 0.35714286 0.37142857 0.38571429 0.4 0.41428571 0.42857143 0.44285714 0.45714286 0.47142857 0.48571429 0.5 0.51428571 0.52857143 0.54285714 0.55714286 0.57142857 0.58571429 0.6 0.61428571 0.62857143 0.64285714 0.65714286 0.67142857 0.68571429 0.7 0.71428571 0.72857143 0.74285714 0.75714286 0.77142857 0.78571429 0.8 0.81428571 0.82857143 0.84285714 0.85714286 0.87142857 0.88571429 0.9 0.91428571 0.92857143 0.94285714 0.95714286 0.97142857 0.98571429 1 1 1 1 1 1
  line L5 (16.4265, -49.9434) -> (16.3148, -49.4692)
  arc A11 (16.3882, -49.3491) -> (16.3148, -49.4692) centre (16.4121, -49.4462) ccw
  arc A12 (16.3882, -49.3491) -> (17.3706, -49.0631) centre (13.5, -37.5997) ccw
  arc A13 (17.497, -49.1249) -> (17.3706, -49.0631) centre (17.4026, -49.1578) ccw
  line L6 (17.497, -49.1249) -> (17.6573, -49.585)
  spline S6 degree 5 poles (17.6573, -49.585) (17.6592, -49.5904) (17.663, -49.601) (17.6692, -49.6168) (17.6781, -49.6376) (17.6903, -49.6631) (17.7033, -49.6884) (17.7167, -49.7134) (17.7304, -49.7384) (17.7442, -49.7633) (17.7582, -49.7882) (17.7725, -49.813) (17.7871, -49.8376) (17.802, -49.8621) (17.8172, -49.8864) (17.8328, -49.9107) (17.8487, -49.9347) (17.8649, -49.9587) (17.8812, -49.9826) (17.8977, -50.0064) (17.9144, -50.0301) (17.9314, -50.0537) (17.9485, -50.0773) (17.9659, -50.1007) (17.9834, -50.124) (18.0012, -50.1472) (18.0192, -50.1704) (18.0374, -50.1934) (18.0557, -50.2164) (18.0743, -50.2393) (18.093, -50.2621) (18.1119, -50.2848) (18.1309, -50.3074) (18.1502, -50.3299) (18.1696, -50.3524) (18.1892, -50.3747) (18.2089, -50.397) (18.2288, -50.4192) (18.2489, -50.4413) (18.2691, -50.4633) (18.2895, -50.4852) (18.31, -50.5071) (18.3307, -50.5289) (18.3515, -50.5506) (18.3725, -50.5722) (18.3937, -50.5937) (18.4149, -50.6152) (18.4364, -50.6365) (18.4579, -50.6578) (18.4797, -50.679) (18.5015, -50.7002) (18.5235, -50.7212) (18.5456, -50.7422) (18.5679, -50.7631) (18.5903, -50.7839) (18.6129, -50.8046) (18.6355, -50.8252) (18.6584, -50.8458) (18.6813, -50.8663) (18.7044, -50.8867) (18.7276, -50.907) (18.7509, -50.9273) (18.7744, -50.9474) (18.7979, -50.9675) (18.8216, -50.9875) (18.8455, -51.0075) (18.8694, -51.0273) (18.8935, -51.0471) (18.9177, -51.0668) (18.942, -51.0864) (18.9665, -51.1059) (18.9861, -51.1215) (19.0009, -51.1331) (19.0108, -51.1409) (19.0158, -51.1447) knots 0 0 0 0 0 0 0.01428571 0.02857143 0.04285714 0.05714286 0.07142857 0.08571429 0.1 0.11428571 0.12857143 0.14285714 0.15714286 0.17142857 0.18571429 0.2 0.21428571 0.22857143 0.24285714 0.25714286 0.27142857 0.28571429 0.3 0.31428571 0.32857143 0.34285714 0.35714286 0.37142857 0.38571429 0.4 0.41428571 0.42857143 0.44285714 0.45714286 0.47142857 0.48571429 0.5 0.51428571 0.52857143 0.54285714 0.55714286 0.57142857 0.58571429 0.6 0.61428571 0.62857143 0.64285714 0.65714286 0.67142857 0.68571429 0.7 0.71428571 0.72857143 0.74285714 0.75714286 0.77142857 0.78571429 0.8 0.81428571 0.82857143 0.84285714 0.85714286 0.87142857 0.88571429 0.9 0.91428571 0.92857143 0.94285714 0.95714286 0.97142857 0.98571429 1 1 1 1 1 1
  arc A14 (19.0158, -51.1447) -> (19.7526, -50.8208) centre (13.5, -37.5997) ccw
  spline S7 degree 5 poles (19.5216, -48.7653) (19.5243, -48.7703) (19.5295, -48.7804) (19.537, -48.7956) (19.5462, -48.8162) (19.5568, -48.8425) (19.5666, -48.8691) (19.5761, -48.8959) (19.5852, -48.9229) (19.5942, -48.9499) (19.6031, -48.9771) (19.6117, -49.0043) (19.62, -49.0317) (19.6279, -49.0593) (19.6356, -49.087) (19.6429, -49.1148) (19.6499, -49.1428) (19.6566, -49.1709) (19.6632, -49.1991) (19.6696, -49.2274) (19.6757, -49.2557) (19.6817, -49.2842) (19.6874, -49.3127) (19.693, -49.3413) (19.6983, -49.37) (19.7034, -49.3989) (19.7083, -49.4278) (19.713, -49.4567) (19.7175, -49.4858) (19.7218, -49.5149) (19.7259, -49.5441) (19.7299, -49.5734) (19.7337, -49.6027) (19.7373, -49.6321) (19.7407, -49.6616) (19.744, -49.6911) (19.747, -49.7207) (19.7499, -49.7504) (19.7526, -49.7801) (19.7552, -49.8099) (19.7576, -49.8398) (19.7598, -49.8697) (19.7619, -49.8996) (19.7638, -49.9296) (19.7655, -49.9597) (19.7671, -49.9899) (19.7685, -50.02) (19.7698, -50.0503) (19.7709, -50.0806) (19.7718, -50.1109) (19.7726, -50.1413) (19.7733, -50.1717) (19.7737, -50.2022) (19.7741, -50.2327) (19.7743, -50.2633) (19.7743, -50.2939) (19.7742, -50.3246) (19.7739, -50.3553) (19.7735, -50.3861) (19.773, -50.4169) (19.7722, -50.4477) (19.7714, -50.4786) (19.7704, -50.5095) (19.7693, -50.5405) (19.768, -50.5715) (19.7665, -50.6025) (19.765, -50.6336) (19.7633, -50.6647) (19.7614, -50.6958) (19.7594, -50.727) (19.7573, -50.7582) (19.7555, -50.7832) (19.7541, -50.802) (19.7531, -50.8145) (19.7526, -50.8208) knots 0 0 0 0 0 0 0.01428571 0.02857143 0.04285714 0.05714286 0.07142857 0.08571429 0.1 0.11428571 0.12857143 0.14285714 0.15714286 0.17142857 0.18571429 0.2 0.21428571 0.22857143 0.24285714 0.25714286 0.27142857 0.28571429 0.3 0.31428571 0.32857143 0.34285714 0.35714286 0.37142857 0.38571429 0.4 0.41428571 0.42857143 0.44285714 0.45714286 0.47142857 0.48571429 0.5 0.51428571 0.52857143 0.54285714 0.55714286 0.57142857 0.58571429 0.6 0.61428571 0.62857143 0.64285714 0.65714286 0.67142857 0.68571429 0.7 0.71428571 0.72857143 0.74285714 0.75714286 0.77142857 0.78571429 0.8 0.81428571 0.82857143 0.84285714 0.85714286 0.87142857 0.88571429 0.9 0.91428571 0.92857143 0.94285714 0.95714286 0.97142857 0.98571429 1 1 1 1 1 1
  line L7 (19.5216, -48.7653) -> (19.2909, -48.3362)
  arc A15 (19.3308, -48.2013) -> (19.2909, -48.3362) centre (19.379, -48.2889) ccw
  arc A16 (19.3308, -48.2013) -> (20.2056, -47.6707) centre (13.5, -37.5997) ccw
  arc A17 (20.3438, -47.6977) -> (20.2056, -47.6707) centre (20.2611, -47.754) ccw
  line L8 (20.3438, -47.6977) -> (20.6177, -48.1007)
  spline S8 degree 5 poles (20.6177, -48.1007) (20.6208, -48.1053) (20.6273, -48.1146) (20.6374, -48.1283) (20.6514, -48.146) (20.6698, -48.1675) (20.6888, -48.1886) (20.7083, -48.2093) (20.7279, -48.2299) (20.7478, -48.2504) (20.7678, -48.2708) (20.7879, -48.291) (20.8084, -48.311) (20.8291, -48.3308) (20.8502, -48.3504) (20.8715, -48.3697) (20.8931, -48.3889) (20.9149, -48.4079) (20.9368, -48.4267) (20.959, -48.4454) (20.9812, -48.464) (21.0037, -48.4825) (21.0264, -48.5007) (21.0492, -48.5189) (21.0722, -48.5369) (21.0954, -48.5547) (21.1188, -48.5724) (21.1423, -48.5899) (21.1659, -48.6074) (21.1898, -48.6247) (21.2137, -48.6418) (21.2379, -48.6589) (21.2621, -48.6758) (21.2865, -48.6926) (21.3111, -48.7092) (21.3358, -48.7258) (21.3606, -48.7422) (21.3856, -48.7585) (21.4107, -48.7746) (21.4359, -48.7907) (21.4613, -48.8066) (21.4868, -48.8224) (21.5124, -48.8381) (21.5381, -48.8536) (21.564, -48.8691) (21.59, -48.8844) (21.6161, -48.8996) (21.6423, -48.9147) (21.6687, -48.9297) (21.6952, -48.9445) (21.7217, -48.9593) (21.7484, -48.9739) (21.7752, -48.9885) (21.8022, -49.0029) (21.8292, -49.0172) (21.8563, -49.0313) (21.8836, -49.0454) (21.9109, -49.0594) (21.9384, -49.0732) (21.966, -49.087) (21.9936, -49.1006) (22.0214, -49.1141) (22.0493, -49.1275) (22.0773, -49.1408) (22.1053, -49.154) (22.1335, -49.1671) (22.1618, -49.1801) (22.1902, -49.1929) (22.2186, -49.2057) (22.2472, -49.2183) (22.2759, -49.2309) (22.2989, -49.2408) (22.3162, -49.2482) (22.3277, -49.2531) (22.3335, -49.2556) knots 0 0 0 0 0 0 0.01428571 0.02857143 0.04285714 0.05714286 0.07142857 0.08571429 0.1 0.11428571 0.12857143 0.14285714 0.15714286 0.17142857 0.18571429 0.2 0.21428571 0.22857143 0.24285714 0.25714286 0.27142857 0.28571429 0.3 0.31428571 0.32857143 0.34285714 0.35714286 0.37142857 0.38571429 0.4 0.41428571 0.42857143 0.44285714 0.45714286 0.47142857 0.48571429 0.5 0.51428571 0.52857143 0.54285714 0.55714286 0.57142857 0.58571429 0.6 0.61428571 0.62857143 0.64285714 0.65714286 0.67142857 0.68571429 0.7 0.71428571 0.72857143 0.74285714 0.75714286 0.77142857 0.78571429 0.8 0.81428571 0.82857143 0.84285714 0.85714286 0.87142857 0.88571429 0.9 0.91428571 0.92857143 0.94285714 0.95714286 0.97142857 0.98571429 1 1 1 1 1 1
  arc A18 (22.3335, -49.2556) -> (22.9614, -48.752) centre (13.5, -37.5997) ccw
  spline S9 degree 5 poles (22.2063, -46.8264) (22.2102, -46.8305) (22.2178, -46.8388) (22.229, -46.8516) (22.2432, -46.8691) (22.2602, -46.8918) (22.2767, -46.9149) (22.2927, -46.9384) (22.3085, -46.9621) (22.3242, -46.9859) (22.3398, -47.0098) (22.3551, -47.0339) (22.3703, -47.0582) (22.3851, -47.0828) (22.3996, -47.1076) (22.4139, -47.1326) (22.4279, -47.1578) (22.4417, -47.1832) (22.4553, -47.2087) (22.4688, -47.2344) (22.4821, -47.2602) (22.4952, -47.2861) (22.5082, -47.3122) (22.5209, -47.3384) (22.5335, -47.3648) (22.5458, -47.3913) (22.558, -47.4179) (22.5701, -47.4447) (22.582, -47.4716) (22.5937, -47.4986) (22.6052, -47.5257) (22.6166, -47.5529) (22.6279, -47.5803) (22.639, -47.6078) (22.6499, -47.6354) (22.6607, -47.663) (22.6713, -47.6909) (22.6818, -47.7188) (22.6921, -47.7468) (22.7023, -47.7749) (22.7123, -47.8031) (22.7222, -47.8314) (22.732, -47.8598) (22.7416, -47.8883) (22.751, -47.9169) (22.7604, -47.9456) (22.7695, -47.9744) (22.7786, -48.0033) (22.7875, -48.0323) (22.7963, -48.0613) (22.8049, -48.0905) (22.8134, -48.1197) (22.8217, -48.149) (22.83, -48.1784) (22.8381, -48.2079) (22.846, -48.2375) (22.8538, -48.2671) (22.8615, -48.2969) (22.8691, -48.3267) (22.8765, -48.3566) (22.8838, -48.3866) (22.891, -48.4166) (22.898, -48.4467) (22.905, -48.4769) (22.9117, -48.5072) (22.9184, -48.5375) (22.9249, -48.568) (22.9313, -48.5984) (22.9376, -48.629) (22.9437, -48.6596) (22.9498, -48.6903) (22.9545, -48.715) (22.9579, -48.7335) (22.9602, -48.7458) (22.9614, -48.752) knots 0 0 0 0 0 0 0.01428571 0.02857143 0.04285714 0.05714286 0.07142857 0.08571429 0.1 0.11428571 0.12857143 0.14285714 0.15714286 0.17142857 0.18571429 0.2 0.21428571 0.22857143 0.24285714 0.25714286 0.27142857 0.28571429 0.3 0.31428571 0.32857143 0.34285714 0.35714286 0.37142857 0.38571429 0.4 0.41428571 0.42857143 0.44285714 0.45714286 0.47142857 0.48571429 0.5 0.51428571 0.52857143 0.54285714 0.55714286 0.57142857 0.58571429 0.6 0.61428571 0.62857143 0.64285714 0.65714286 0.67142857 0.68571429 0.7 0.71428571 0.72857143 0.74285714 0.75714286 0.77142857 0.78571429 0.8 0.81428571 0.82857143 0.84285714 0.85714286 0.87142857 0.88571429 0.9 0.91428571 0.92857143 0.94285714 0.95714286 0.97142857 0.98571429 1 1 1 1 1 1
  line L9 (22.2063, -46.8264) -> (21.8724, -46.4716)
  arc A19 (21.876, -46.3309) -> (21.8724, -46.4716) centre (21.9452, -46.4031) ccw
  arc A20 (21.876, -46.3309) -> (22.5837, -45.592) centre (13.5, -37.5997) ccw
  arc A21 (22.7241, -45.5824) -> (22.5837, -45.592) centre (22.6588, -45.6581) ccw
  line L10 (22.7241, -45.5824) -> (23.093, -45.9007)
  spline S10 degree 5 poles (23.093, -45.9007) (23.0973, -45.9044) (23.1059, -45.9116) (23.1191, -45.9222) (23.1373, -45.9357) (23.1606, -45.9518) (23.1845, -45.9672) (23.2086, -45.9822) (23.233, -45.997) (23.2574, -46.0116) (23.282, -46.0261) (23.3067, -46.0405) (23.3317, -46.0545) (23.3568, -46.0683) (23.3822, -46.0817) (23.4078, -46.0949) (23.4336, -46.1078) (23.4596, -46.1205) (23.4857, -46.133) (23.5119, -46.1454) (23.5382, -46.1575) (23.5647, -46.1695) (23.5913, -46.1813) (23.618, -46.1929) (23.6449, -46.2044) (23.6719, -46.2156) (23.6991, -46.2266) (23.7264, -46.2375) (23.7537, -46.2482) (23.7812, -46.2587) (23.8088, -46.2691) (23.8365, -46.2794) (23.8643, -46.2894) (23.8923, -46.2993) (23.9203, -46.309) (23.9484, -46.3186) (23.9767, -46.328) (24.005, -46.3373) (24.0334, -46.3464) (24.0619, -46.3554) (24.0906, -46.3642) (24.1193, -46.3728) (24.1481, -46.3814) (24.177, -46.3897) (24.206, -46.398) (24.235, -46.406) (24.2642, -46.414) (24.2934, -46.4218) (24.3228, -46.4294) (24.3522, -46.4369) (24.3817, -46.4443) (24.4112, -46.4515) (24.4409, -46.4586) (24.4706, -46.4656) (24.5004, -46.4724) (24.5303, -46.479) (24.5603, -46.4856) (24.5903, -46.492) (24.6204, -46.4983) (24.6506, -46.5044) (24.6809, -46.5104) (24.7112, -46.5163) (24.7416, -46.522) (24.7721, -46.5276) (24.8026, -46.5331) (24.8332, -46.5384) (24.8639, -46.5436) (24.8946, -46.5487) (24.9254, -46.5537) (24.9563, -46.5585) (24.9872, -46.5632) (25.012, -46.5668) (25.0306, -46.5695) (25.0431, -46.5713) (25.0493, -46.5722) knots 0 0 0 0 0 0 0.01428571 0.02857143 0.04285714 0.05714286 0.07142857 0.08571429 0.1 0.11428571 0.12857143 0.14285714 0.15714286 0.17142857 0.18571429 0.2 0.21428571 0.22857143 0.24285714 0.25714286 0.27142857 0.28571429 0.3 0.31428571 0.32857143 0.34285714 0.35714286 0.37142857 0.38571429 0.4 0.41428571 0.42857143 0.44285714 0.45714286 0.47142857 0.48571429 0.5 0.51428571 0.52857143 0.54285714 0.55714286 0.57142857 0.58571429 0.6 0.61428571 0.62857143 0.64285714 0.65714286 0.67142857 0.68571429 0.7 0.71428571 0.72857143 0.74285714 0.75714286 0.77142857 0.78571429 0.8 0.81428571 0.82857143 0.84285714 0.85714286 0.87142857 0.88571429 0.9 0.91428571 0.92857143 0.94285714 0.95714286 0.97142857 0.98571429 1 1 1 1 1 1
  arc A22 (25.0493, -46.5722) -> (25.5254, -45.9232) centre (13.5, -37.5997) ccw